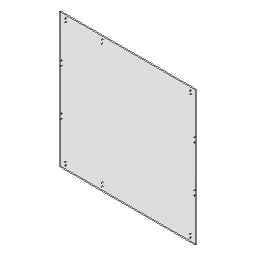
enclosure-side250 v17 (Autodesk Fusion 360 design; units mm, degrees)
Autodesk Fusion 360 part; units mm, degrees
sketch "Sketch1" plane through (0, 0, 0) normal (0, 0, 1) x (1, 0, 0)
  line L0 (298.2, -291.299) -> (-298.2, -291.299)
  line L1 (-298.2, -291.299) -> (-298.2, 291.299)
  line L2 (-298.2, 291.299) -> (298.2, 291.299)
  line L3 (298.2, 291.299) -> (298.2, -291.299)
  line L4 (298.2, -291.299) -> (-298.2, 291.299) construction
  line L5 (-298.2, -291.299) -> (298.2, 291.299) construction
  line L6 (-275.35, 291.299) -> (-275.35, -291.299) construction
  circle A0 centre (-275.35, 280.639) radius 2
  circle A1 centre (-275.35, 266.5) radius 2
  circle A2 centre (-275.35, -280.639) radius 2
  circle A3 centre (-275.35, -266.5) radius 2
  line L7 (275.35, 291.299) -> (275.35, -291.299) construction
  circle A4 centre (275.35, 280.639) radius 2
  circle A5 centre (275.35, 266.5) radius 2
  circle A6 centre (275.35, -280.639) radius 2
  circle A7 centre (275.35, -266.5) radius 2
  line L8 (-275.35, -266.5) -> (275.35, -266.5) construction
  circle A8 centre (-114.4, -266.5) radius 2
  line L9 (-114.4, -291.299) -> (-114.4, 278.639) construction
  circle A9 centre (-114.4, 266.5) radius 2
  circle A10 centre (-114.4, 280.639) radius 2
  circle A11 centre (-114.4, -280.639) radius 2
  line L10 (-298.2, 296.299) -> (298.2, 296.299)
  line L11 (298.2, 296.299) -> (298.2, -296.299)
  line L12 (298.2, -296.299) -> (-298.2, -296.299)
  line L13 (-298.2, -296.299) -> (-298.2, 296.299)
  line L14 (-298.2, 101.299) -> (298.2, 101.299) construction
  line L15 (-298.2, -101.299) -> (298.2, -101.299) construction
  circle A12 centre (293.2, -91.299) radius 2
  circle A13 centre (293.2, -111.299) radius 2
  circle A14 centre (293.2, 91.299) radius 2
  circle A15 centre (293.2, 111.299) radius 2
  circle A16 centre (-293.2, 111.299) radius 2
  circle A17 centre (-293.2, 91.299) radius 2
  circle A18 centre (-293.2, -91.299) radius 2
  circle A19 centre (-293.2, -111.299) radius 2
  line L16 (-275.35, 266.5) -> (275.35, 266.5) construction
  line L17 (-275.35, 280.639) -> (275.35, 280.639) construction
  line L18 (275.35, -280.639) -> (-275.35, -280.639) construction
  dimension "d1" = 596.4
  dimension "d2" = 582.598
  dimension "d3" = 22.85
  dimension "d4" = 4
  dimension "d6" = 4
  dimension "d8" = 4
  dimension "d9" = 4
  dimension "d12" = 22.85
  dimension "d13" = 4
  dimension "d14" = 4
  dimension "d17" = 4
  dimension "d18" = 4
  dimension "d21" = 4
  dimension "d22" = 4
  dimension "d23" = 4
  dimension "d24" = 4
  dimension "d29" = 5
  dimension "d31" = 5
  dimension "d38" = 190
  dimension "d39" = 190
  dimension "d40" = 4
  dimension "d41" = 4
  dimension "d42" = 10
  dimension "d43" = 10
  dimension "d44" = 5
  dimension "d45" = 5
  dimension "d46" = 4
  dimension "d47" = 4
  dimension "d48" = 10
  dimension "d49" = 10
  dimension "d50" = 5
  dimension "d51" = 5
  dimension "d52" = 4
  dimension "d53" = 4
  dimension "d54" = 5
  dimension "d55" = 5
  dimension "d56" = 10
  dimension "d57" = 10
  dimension "d58" = 4
  dimension "d59" = 4
  dimension "d60" = 5
  dimension "d61" = 5
  dimension "d62" = 10
  dimension "d63" = 10
  dimension "d70" = 24.799
  dimension "d71" = 10.66
  dimension "d72" = 10.66
  dimension "d73" = 24.799
  dimension "d74" = 412.6
  measures "d3" distance of L1 L6
  measures "d4" diameter of A0
  measures "d6" diameter of A1
  measures "d8" diameter of A2
  measures "d9" diameter of A3
  measures "d12" distance of L3 L7
  measures "d13" diameter of A4
  measures "d14" diameter of A5
  measures "d17" diameter of A6
  measures "d18" diameter of A7
  measures "d21" diameter of A8
  measures "d22" diameter of A9
  measures "d23" diameter of A10
  measures "d24" diameter of A11
  measures "d29" distance of L2 L10
  measures "d31" distance of L0 L12
  measures "d38" distance of L2 L14
  measures "d39" distance of L0 L15
  measures "d40" diameter of A12
  measures "d41" diameter of A13
  measures "d46" diameter of A14
  measures "d47" diameter of A15
  measures "d52" diameter of A16
  measures "d53" diameter of A17
  measures "d58" diameter of A18
  measures "d59" diameter of A19
  measures "d70" distance of L2 L16
  measures "d71" distance of L2 L17
  measures "d72" distance of L0 L18
  measures "d73" distance of L0 L8
  measures "d74" distance of L9 L11
extrude "Extrude1" add sketch "Sketch1" along normal blind 5 makes body 1
copy_body "Body->Comp1" bodies 1 removing the originals makes body 2 in component "Side"
component "Side" placed x (1, 0, 0) y (0, 1, 0) z (0, 0, 1) at (0, 0, 0)
equation "d1 = YRailLength + 246.4 mm"
equation "d2 = PrintHeight + 282.598 mm"
equation "d29 = WallThickness"
equation "d31 = WallThickness"
equation "WallThickness = 5 mm"
equation "YRailLength = 350 mm"
equation "PrintHeight = 300 mm"
equation "d74 = YRailLength + 62.6 mm"
named bodies: "Side"
